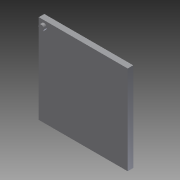
# Autodesk Inventor part: lasiness
Saved by Autodesk Inventor 2011 (Build 150239000, 239)
## iProperties
Created: 2011-07-09
Part Number: lasiness
Document SubType Name: Modeling
Designer: adowning
Density: 1 g/cm^3
Author: adowning
Autodesk Inventor part; units mm, degrees
ref_plane "YZ Plane" through (0, 0, 0) normal (1, 0, 0) x (0, 1, 0)
ref_plane "XZ Plane" through (0, 0, 0) normal (0, 1, 0) x (-1, 0, 0)
ref_plane "XY Plane" through (0, 0, 0) normal (0, 0, 1) x (1, 0, 0)
sketch "Sketch1" plane through (0, 0, 0) normal (0, 0, 1) x (1, 0, 0)
  line L0 (-24.4308, 23.0298) -> (77.1692, 23.0298)
  line L1 (77.1692, 23.0298) -> (77.1692, -78.5702)
  line L2 (77.1692, -78.5702) -> (-24.4308, -78.5702)
  line L3 (-24.4308, -78.5702) -> (-24.4308, 23.0298)
  point P0 (0, 0)
  dimension "d0" = 101.6
  dimension "d1" = 101.6
  constraints: 8 end point, 2 parallel, 1 horizontal, 1 perpendicular
  measures "d0" distance of L1.end L2.end
  measures "d1" distance of L0.end L1.end
extrude "Extrusion1" add sketch "Sketch1" along normal blind 6.35
sketch "Sketch2" plane through (0, 0, 6.35) normal (0, 0, 1) x (1, 0, 0)
  line L0 (-24.4308, 23.0298) -> (26.3692, 23.0298)
  line L1 (26.3692, 23.0298) -> (26.3692, -27.7702)
  line L2 (26.3692, -27.7702) -> (-24.4308, -27.7702)
  line L3 (-24.4308, -27.7702) -> (-24.4308, 23.0298)
  circle A0 centre (26.3692, -27.7702) radius 12.7
  point P0 (0, 0)
  dimension "d4" = 50.8
  dimension "d5" = 50.8
  dimension "d6" = 25.4
  constraints: 8 end point, 2 parallel, 1 centre point, 1 coincident, 1 horizontal, 1 perpendicular
  measures "d4" distance of L1.end L2.end
  measures "d5" distance of L0.end L1.end
  measures "d6" diameter of A0
extrude "Extrusion2" cut sketch "Sketch2" against normal blind 6.35 contours A0 L2 L1 | L1 L2 A0
sketch "Sketch3" plane through (0, 0, 6.35) normal (0, 0, 1) x (1, 0, 0)
  line L0 (-24.4308, 23.0298) -> (77.1692, 23.0298) projected
  line L1 (-24.4308, -78.5702) -> (-24.4308, 23.0298) projected
  line L2 (-24.4308, 23.0298) -> (-24.4308, -27.7702)
  line L3 (-24.4308, -27.7702) -> (-24.4308, 11.9935)
  line L4 (-24.4308, 11.9935) -> (-13.3818, 11.9935)
  line L5 (-13.3818, 11.9935) -> (-13.3818, 23.0298)
  line L6 (-13.3818, 23.0298) -> (-24.4308, 23.0298)
  line L7 (-24.4308, 23.0298) -> (-24.4308, 11.9935)
  circle A0 centre (-13.3818, 11.9935) radius 3.175
  point P0 (0, 0)
  dimension "d9" = 50.8
  dimension "d10" = 39.7637
  dimension "d11" = 11.049
  dimension "d12" = 6.35
  constraints: 12 end point, 2 parallel, 2 point on line, 1 centre point, 1 coincident, 1 horizontal, 1 midpoint, 1 perpendicular
  measures "d9" distance of L0.start L2.end
  measures "d10" distance of L2.end L3.end
  measures "d11" distance of L6.end L5.end
  measures "d12" diameter of A0
extrude "Extrusion3" add sketch "Sketch3" along normal blind 6.35 contours A0 L4 L5 | L5 L4 A0
sketch "Sketch4" plane through (0, 0, 6.35) normal (0, 0, 1) x (1, 0, 0)
  circle A0 centre (26.3692, -27.7702) radius 12.7 projected
  point P0 (0, 0)
extrude "Extrusion4" add sketch "Sketch4" against normal blind 19.05
sketch "Sketch5" plane through (0, 0, 6.35) normal (0, 0, 1) x (1, 0, 0)
  line L0 (-24.4308, -78.5702) -> (-24.4308, 23.0298) projected
  line L1 (-24.4308, 23.0298) -> (-24.4308, -27.7702)
  line L2 (-24.4308, -27.7702) -> (-24.4308, 17.0735)
  line L3 (-24.4308, 23.0298) -> (-18.4618, 23.0298)
  line L4 (-18.4618, 23.0298) -> (-18.4618, 17.0735)
  line L5 (-18.4618, 17.0735) -> (-24.4308, 17.0735)
  line L6 (-24.4308, 17.0735) -> (-24.4308, 23.0298)
  circle A0 centre (-18.4618, 17.0735) radius 3.175
  point P0 (0, 0)
  dimension "d17" = 50.8
  dimension "d18" = 44.8437
  dimension "d19" = 5.969
  dimension "d20" = 6.35
  constraints: 12 end point, 2 parallel, 1 centre point, 1 coincident, 1 horizontal, 1 midpoint, 1 perpendicular, 1 point on line
  measures "d17" distance of L0.end L1.end
  measures "d18" distance of L1.end L2.end
  measures "d19" distance of L4.end L5.end
  measures "d20" diameter of A0
extrude "Extrusion5" add sketch "Sketch5" along normal blind 3.175 contours A0 L4 L5 | L5 L4 A0
sketch "Sketch6" plane through (-13.3818, 11.9935, 12.7) normal (0, 0, 1) x (1, 0, 0)
  circle A0 centre (0, 0) radius 3.175 projected
  point P0 (13.3818, -11.9935)
extrude "Extrusion6" cut sketch "Sketch6" against normal blind 6.35
body "Solid1"
